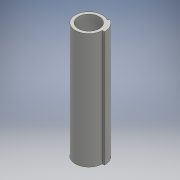
# Autodesk Inventor part: Drum
Saved by Autodesk Inventor 2016 (Build 200138000, 138)
## iProperties
Created: 2016-12-01
Part Number: Drum
Material: Generic
Document SubType Name: Modeling
Designer: Kevin
Density: 1 g/cm^3
Appearance: Default
Author: Kevin
Autodesk Inventor part; units mm, degrees
ref_plane "YZ Plane" through (0, 0, 0) normal (1, 0, 0) x (0, 1, 0)
ref_plane "XZ Plane" through (0, 0, 0) normal (0, 1, 0) x (-1, 0, 0)
ref_plane "XY Plane" through (0, 0, 0) normal (0, 0, 1) x (1, 0, 0)
sketch "Sketch1" plane through (0, 0, 0) normal (0, 0, 1) x (1, 0, 0)
  circle A0 centre (0, 0) radius 57.15
  circle A1 centre (0, 0) radius 44.45
  line L0 (57.15, 0) -> (66.675, 0)
  arc A2 (66.675, 0) -> (33.3375, 57.7422) centre (0, 0) ccw
  line L1 (0, 0) -> (33.3375, 57.7422) construction
  line L2 (0, 0) -> (66.675, 0) construction
  line L3 (28.575, 49.4934) -> (33.3375, 57.7422)
  dimension "d0" = 114.3
  dimension "d2" = 88.9
  dimension "d4" = 60
  constraints: 8 end point, 4 point on circle, 3 centre point, 2 coincident, 1 collinear, 1 horizontal, 1 point on line
  measures "d0" diameter of A0
  measures "d2" diameter of A1
  measures "d4" angle of L2 L1
extrude "Extrusion1" add sketch "Sketch1" along normal blind 491.25
body "Solid1"
